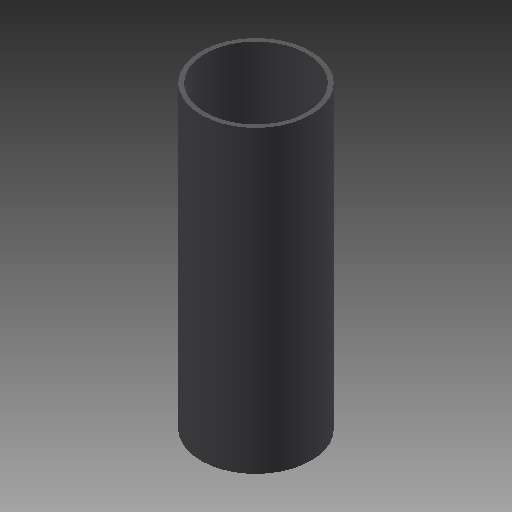
# Autodesk Inventor part: 042.212-FO1_BM_tube
Saved by Autodesk Inventor 2017 (Build 210142000, 142)
## iProperties
Category: PARTsolutions
Company: BIMBA
Created: 2017-01-25
Part Number: 042.212-FO1_BM_tube
Catalog Web Link: www.cadenas.de
Description: FO1_basic_model_tube-Bimba FLAT-1
Vendor: BIMBA
Document SubType Name: Modeling
Designer: psAdmin
Manufacturer: BIMBA
Mass: 2.75708 g
Surface Area: 71.0113 cm^2
Volume: 2.75708 cm^3
Density: 1 g/cm^3
Material: Generic
Appearance: PSOLRGB-180-180-180
PSOL_IDENT_0: {$CADENAS_DATA\23d-libs\bimba\bimba\bimba_imperial\bimba_full_line\flat_cylinders\fo1\fo1_basic_mode
PSOL_IDENT_1: l_tube.prj},203 {VTYP=3D},{NB=042.212-FO1_BM_tube},{LINA=042.212-FO1_BM_tube},{NN=FO1_basic_model_tu
PSOL_IDENT_2: be},{DATE=01.12.2016 06:16:11},{GEOMDATE=25.05.2016 11:19:00},{VERSION=},{LINEID=20},{LINESUBID=-1},
PSOL_IDENT_3: {WBVAR=STROKE,AB}  {NB=042.212-FO1_BM_tube},{LINA=042.212-FO1_BM_tube},{KT=DUMMY},{PN=042.212-FO1_BM
PSOL_IDENT_4: _tube},{BORE=0.75000000},{BOREPN=04},{STROKE=2.21200},{STROKEMIN=0.34},{AB=},{A=1.50000000},{BA=0.56
PSOL_IDENT_5: 000},{BB=0.69000},{BC=1.94},{BD=2.19},{C=1.22000000},{DD=4.00000000},{D=0.13800000},{CPIL=0.15600000
PSOL_IDENT_6: },{DC=0.23500000},{DCP=0.14800000},{DCD=1.21800000},{ES=0.19000000},{EC=0.19000000},{ED=0.46000000},
PSOL_IDENT_7: {F=0.31000000},{H=0.25000000},{J=0.34000000},{K=0.14000000},{L=0.19000000},{LDP=0.12600000},{LP=0.12
PSOL_IDENT_8: 500000},{LPDP=0.44000000},{TD=0.80500000},{TDDP=0.17000},{TD1=0.80000},{TD2=0.81200},{TDIN=0.75000},
PSOL_IDENT_9: {LSF=0.31250000},{LSFDP=0.02000000},{BC1=0.81000},{BC2=1.38000},{BC3=1.94000},{BC4=2.50000},{BD1=1.0
PSOL_IDENT_10: 6000},{BD2=1.62000},{BD3=2.19000},{BD4=2.75000},{TDAB=0.874},{TDA=0.812}
NN: FO1_basic_model_tube
NT: Bimba FLAT-1
NB: 042.212-FO1_BM_tube
NBSYN: $PN.
LINA: 042.212-FO1_BM_tube
PN: 042.212-FO1_BM_tube
BORE: 3/4
BOREPN: 04
STROKE: 2.21200
AB: Standard
A: 1.50000000
BA: 0.56000
BB: 0.69000
C: 1.22000000
DD: 4.00000000
D: 0.13800000
CPIL: 0.15600000
DC: 0.23500000
DCP: 0.14800000
DCD: 1.21800000
ES: 0.19000000
EC: 0.19000000
ED: 0.46000000
F: 0.31000000
H: 0.25000000
J: 0.34000000
K: 0.14000000
L: 0.19000000
LDP: 0.12600000
LP: 0.12500000
LPDP: 0.44000000
TD: 0.80500000
TDDP: 0.17000
TD1: 0.80000
TD2: 0.81200
TDIN: 0.75000
LSF: 0.31250000
LSFDP: 0.02000000
BC1: 0.81000
BC2: 1.38000
BC3: 1.94000
BC4: 2.50000
BD1: 1.06000
BD2: 1.62000
BD3: 2.19000
BD4: 2.75000
TDAB: 0.874
SUPPLIER: BIMBA
ARTICLENO: 042.212-FO1_BM_tube
BOMINFO: 042.212-FO1_BM_tube
CREATOR: CADENAS GmbH
Title: 042.212-FO1_BM_tube
Author: Cadenas PARTsolutions
Comments: Bimba FLAT-1
Autodesk Inventor part; units mm, degrees
sketch "Sketch_4" plane through (0, 0, 0) normal (0, 0, 1) x (1, 0, 0)
  line L0 (0, 0) -> (0, 56.1848)
  line L1 (9.525, 56.1848) -> (9.525, 0)
  line L2 (9.525, 0) -> (10.3124, 0)
  line L3 (10.3124, 0) -> (10.3124, 56.1848)
  line L4 (10.3124, 56.1848) -> (9.525, 56.1848)
  constraints: 10 end point
revolve "Revolution1" add sketch "Sketch_4" angle 360 about axis through (0, 0, 0) along (0, -1, 0)
ref_plane "tube_rear_XY" through (0, 56.1848, 0) normal (0, 1, 0) x (1, 0, 0)
ref_plane "tube_rear_YZ" through (0, 56.1848, 0) normal (1, 0, 0) x (0, 0, -1)
ref_plane "tube_rear_ZX" through (0, 56.1848, 0) normal (0, 0, -1) x (0, 1, 0)
ref_plane "tube_rod_guide_XY" through (0, 0, 0) normal (0, 1, 0) x (1, 0, 0)
ref_plane "tube_rod_guide_YZ" through (0, 0, 0) normal (1, 0, 0) x (0, 0, -1)
ref_plane "tube_rod_guide_ZX" through (0, 0, 0) normal (0, 0, -1) x (0, 1, 0)
body "Solid1"
